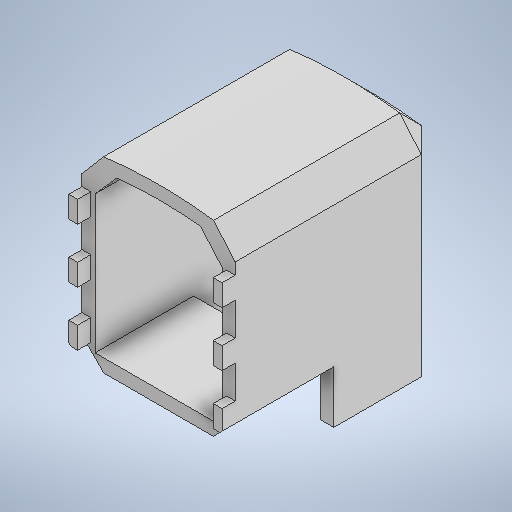
# Autodesk Inventor part: thermal camera lid
Saved by Autodesk Inventor 2025.2 (Build 292293000, 293)
## iProperties
Created: 2025-08-14
Part Number: thermal camera lid
Material: Generic
Document SubType Name: Modeling
Designer: mateo
Density: 1 g/cm^3
Appearance: Default
Author: mateo
Autodesk Inventor part; units mm, degrees
ref_plane "YZ Plane" through (0, 0, 0) normal (1, 0, 0) x (0, 1, 0)
ref_plane "XZ Plane" through (0, 0, 0) normal (0, 1, 0) x (-1, 0, 0)
ref_plane "XY Plane" through (0, 0, 0) normal (0, 0, 1) x (1, 0, 0)
sketch "Sketch1" plane through (0, 0, 0) normal (0, 0, 1) x (1, 0, 0)
  line L0 (-35, -117.7273) -> (-35, -195.6818)
  line L1 (-35, -195.6818) -> (35, -195.6818)
  line L2 (35, -195.6818) -> (35, -117.7273)
  arc A0 (35, -117.7273) -> (-35, -117.7273) centre (0, -308.6364) ccw
  point P0 (0, 0)
  dimension "d46" = 70
  constraints: 6 end point, 2 point on circle, 1 centre point, 1 parallel
  measures "d46" distance of L0.end L1.end
extrude "Extrusion1" add sketch "Sketch1" along normal blind 95
sketch "Sketch9" plane through (35, -195.6818, 0) normal (1, 0, 0) x (0, 0, -1)
  line L0 (0, 0) -> (-50, 0)
  line L1 (-50, 0) -> (-50, -20)
  line L2 (-50, -20) -> (0, -20)
  line L3 (0, -20) -> (0, 0)
  line L4 (0, 0) -> (-95, 0) projected
  point P0 (0, 195.6818)
  dimension "d41" = 50
  dimension "d70" = 20
  dimension "d71" = 0
  constraints: 8 end point, 2 parallel, 1 collinear, 1 horizontal, 1 perpendicular
  measures "d41" distance of L2.end L1.end
  measures "d70" distance of L2.end L0.start
  measures "d71" distance between parallel lines of L4 L0
extrude "Extrusion7" add sketch "Sketch9" against normal blind 70
shell "Shell3" thickness 6 removed faces 4 at (11.6667, -202.3485, 50) at (11.6667, -195.6818, 80) at (0, -168.6364, 95) at (11.6667, -215.6818, 33.3333)
chamfer "Chamfer3" distance 10 angle 45 5 edges at (0, -114.5455, 0) (35, -117.7273, 47.5) (35, -166.7045, 0) (-35, -117.7273, 47.5) (-35, -166.7045, 0)
chamfer "Chamfer4" distance 10 angle 45 5 edges at (29, -169.2382, 6) (29, -122.7945, 50.5) (0, -120.5455, 6) (-29, -169.2382, 6) (-29, -122.7945, 50.5)
sketch "Sketch10" plane through (0, 0, 95) normal (0, 0, 1) x (1, 0, 0)
  line L0 (-35, -129.3148) -> (-35, -202.7975)
  line L1 (-35, -132.9423) -> (-31, -132.9423)
  line L2 (-31, -132.9423) -> (-31, -142.8423)
  line L3 (-31, -142.8423) -> (-35, -142.8423)
  line L4 (-35, -142.8423) -> (-35, -132.9423)
  line L5 (-31, -167.7423) -> (-35, -167.7423)
  line L6 (-31, -157.8423) -> (-31, -167.7423)
  line L7 (-35, -167.7423) -> (-35, -157.8423)
  line L8 (-35, -157.8423) -> (-31, -157.8423)
  line L9 (-31, -192.6423) -> (-35, -192.6423)
  line L10 (-31, -182.7423) -> (-31, -192.6423)
  line L11 (-35, -192.6423) -> (-35, -182.7423)
  line L12 (-35, -182.7423) -> (-31, -182.7423)
  line L13 (29, -130.0108) -> (29, -200.8368)
  line L14 (0, -182.3424) -> (0, -129.0148) construction
  ellipse E0 centre (0, -136.525) end of major axis (3.5, -136.525) minor radius 1.589
  line L15 (-29, -200.8368) -> (-29, -130.0108)
  line L16 (29, -200.8368) -> (29, -130.0108)
  line L17 (35, -132.9423) -> (31, -132.9423)
  line L18 (31, -132.9423) -> (31, -142.8423)
  line L19 (35, -142.8423) -> (35, -132.9423)
  line L20 (31, -142.8423) -> (35, -142.8423)
  line L21 (35, -182.7423) -> (31, -182.7423)
  line L22 (31, -182.7423) -> (31, -192.6423)
  line L23 (31, -192.6423) -> (35, -192.6423)
  line L24 (35, -192.6423) -> (35, -182.7423)
  line L25 (31, -167.7423) -> (35, -167.7423)
  line L26 (31, -157.8423) -> (31, -167.7423)
  line L27 (35, -167.7423) -> (35, -157.8423)
  line L28 (35, -157.8423) -> (31, -157.8423)
  line L29 (35, -195.6818) -> (35, -127.7273) projected
  line L30 (35, -127.7273) -> (31.2472, -127.7273)
  point P0 (0, 0)
  point P1 (90.961, -350.6639)
  point P2 (236.5575, 17.4343)
  point P3 (236.5575, 2.4343)
  point P4 (236.5575, -7.5657)
  point P5 (236.5575, -22.5657)
  point P6 (236.5575, -32.5657)
  dimension "d54" = 9.9
  dimension "d55" = 9.9
  dimension "d56" = 9.9
  dimension "d57" = 15
  dimension "d58" = 15
  dimension "d59" = 29
  dimension "d60" = 29
  constraints: 60 end point, 12 symmetric about line, 6 parallel, 4 horizontal, 3 perpendicular, 1 centre point, 1 line through centre, 1 point on line
  measures "d54" distance of L1.end L2.end
  measures "d55" distance of L6.start L5.start
  measures "d56" distance of L10.start L9.start
  measures "d57" distance between parallel lines of L5 L12
  measures "d58" distance between parallel lines of L3 L8
  measures "d59" distance between parallel lines of L15 L14
  measures "d60" distance between parallel lines of L13 L14
extrude "Extrusion8" add sketch "Sketch10" along normal blind 6 contours L1 L2 L3 L0 | L8 L6 L5 L0 | L12 L10 L9 L0 | L19 L20 L18 L17 | L24 L23 L22 L21 | L26 L28 L27 L25
sketch "Sketch11" plane through (35, -215.6818, 50) normal (1, 0, 0) x (0, 0, -1)
  line L0 (0, 20) -> (-45, 20) projected
  line L1 (0, 20) -> (-45, 20)
  line L2 (-45, 20) -> (-45, 14)
  line L3 (-45, 14) -> (0, 14)
  line L4 (0, 14) -> (0, 20)
  point P0 (50, 215.6818)
  point P1 (-45, 20)
  dimension "d64" = 6
  constraints: 8 end point, 2 parallel, 1 horizontal, 1 perpendicular
  measures "d64" distance of L2.end L1.end
extrude "Extrusion9" add sketch "Sketch11" against normal blind 70
chamfer "Chamfer5" distance 10 angle 45 2 edges at (35, -201.6818, 72.5) (-35, -201.6818, 72.5)
body "Solid1"
